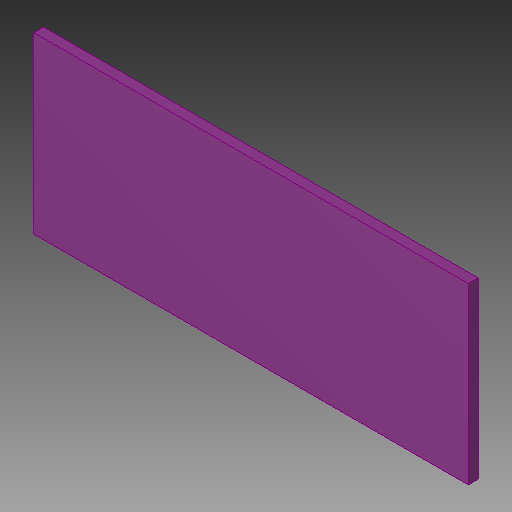
# Autodesk Inventor part: ARDUINO-NANO-3_0
Saved by Autodesk Inventor 2019 (Build 230136000, 136)
## iProperties
Created: 2019-10-02
Part Number: ARDUINO-NANO-3_0
Material: Generic
Document SubType Name: Modeling
Designer: rybit
Density: 1 g/cm^3
Appearance: ARDUINO-NANO-3_0, ARDUINO-NANO-3_0
Author: rybit
Autodesk Inventor part; units mm, degrees
ref_plane "YZ Plane" through (0, 0, 0) normal (1, 0, 0) x (0, 1, 0)
ref_plane "XZ Plane" through (0, 0, 0) normal (0, 1, 0) x (-1, 0, 0)
ref_plane "XY Plane" through (0, 0, 0) normal (0, 0, 1) x (1, 0, 0)
sketch "ARDUINO-NANO-3_0, ARDUINO-NANO-3_0_10" plane through (0, 0, 0) normal (0, 0, 1) x (1, 0, 0)
  line L0 (-22.86, 8.9535) -> (21.59, 8.9535)
  line L1 (21.59, 8.9535) -> (21.59, -8.89)
  line L2 (21.59, -8.89) -> (-22.86, -8.89)
  line L3 (-22.86, -8.89) -> (-22.86, 8.9535)
  constraints: 8 end point
extrude "Extrusion1" add sketch "ARDUINO-NANO-3_0, ARDUINO-NANO-3_0_10" along normal blind 1
body "Solid1"
